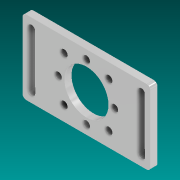
# Autodesk Inventor part: mounting plate stepper motor base 4 mm
Saved by Autodesk Inventor 2020.3 (Build 243373000, 373)
## iProperties
Created: 2020-05-15
Part Number: mounting plate stepper motor base 4 mm
Material: Aluminum 6061
Document SubType Name: Modeling
Designer: Svend
Density: 2.7 g/cm^3
Appearance: Aluminum - Polished
Author: Svend
Autodesk Inventor part; units mm, degrees
ref_plane "YZ Plane" through (0, 0, 0) normal (1, 0, 0) x (0, 1, 0)
ref_plane "XZ Plane" through (0, 0, 0) normal (0, 1, 0) x (-1, 0, 0)
ref_plane "XY Plane" through (0, 0, 0) normal (0, 0, 1) x (1, 0, 0)
sketch "Sketch1" plane through (0, 0, 0) normal (0, 0, 1) x (1, 0, 0)
  circle A0 centre (0, 0) radius 21
  circle A1 centre (16, 0) radius 2
  circle A2 centre (0, 16) radius 2
  circle A3 centre (-16, 0) radius 2
  circle A4 centre (0, -16) radius 2
  line L0 (-14.8492, -14.8492) -> (14.8492, 14.8492)
  line L1 (0, -21) -> (0, 21)
  circle A5 centre (11.3137, 11.3137) radius 1.5
  circle A6 centre (0, 0) radius 12.6
  line L2 (-36.25, -21) -> (36.25, -21)
  line L3 (36.25, 21) -> (-36.25, 21)
  line L4 (-21, -21) -> (21, 21) construction
  line L5 (21, -21) -> (-21, 21) construction
  line L6 (-36.25, 21) -> (-36.25, -21)
  line L7 (36.25, 21) -> (36.25, -21)
  line L8 (-33.35, 17.5) -> (-29.15, 17.5)
  line L9 (-29.15, 17.5) -> (-29.15, -17.5)
  line L10 (-29.15, -17.5) -> (-33.35, -17.5)
  line L11 (-33.35, -17.5) -> (-33.35, 17.5)
  line L12 (-33.35, 17.5) -> (-29.15, -17.5) construction
  line L13 (-29.15, 17.5) -> (-33.35, -17.5) construction
  line L14 (29.15, 17.5) -> (33.35, 17.5)
  line L15 (33.35, 17.5) -> (33.35, -17.5)
  line L16 (33.35, -17.5) -> (29.15, -17.5)
  line L17 (29.15, -17.5) -> (29.15, 17.5)
  line L18 (29.15, 17.5) -> (33.35, -17.5) construction
  line L19 (33.35, 17.5) -> (29.15, -17.5) construction
  line L20 (-26.25, 21) -> (-26.25, -21)
  line L21 (26.25, 21) -> (26.25, -21)
  circle A7 centre (-12.7279, -12.7279) radius 1.621 projected
  circle A8 centre (0, 0) radius 12.5 projected
  circle A9 centre (-12.7279, -12.7279) radius 2 projected
  circle A10 centre (12.7279, 12.7279) radius 2 projected
  circle A11 centre (-12.7279, 12.7279) radius 2 projected
  circle A12 centre (12.7279, -12.7279) radius 2 projected
  circle A13 centre (16, 0) radius 1.6 projected
  circle A14 centre (-16, 0) radius 1.6 projected
  circle A15 centre (0, 16) radius 1.6 projected
  circle A16 centre (0, -16) radius 1.6 projected
  circle A17 centre (0, 0) radius 20.7 projected
  point P0 (-18.984, 8.9782)
  point P1 (-18.984, -8.9782)
  point P2 (-31.25, 0)
  point P3 (31.25, 0)
  point P4 (-31.25, 0)
  point P5 (31.25, 0)
  point P6 (31.25, 0)
  point P7 (31.25, 21)
  point P8 (-31.25, 0)
  point P9 (-31.25, 21)
  point P10 (31.25, 21)
  point P11 (0, 21)
  point P12 (0, -21)
  dimension "d0" = 42
  dimension "d1" = 4
  dimension "d5" = 16
  dimension "d8" = 360
  dimension "d10" = 45
  dimension "d11" = 3
  dimension "d12" = 16
  dimension "d19" = 25.2
  dimension "d31" = 4.2
  dimension "d32" = 35
  dimension "d33" = 4.2
  dimension "d38" = 5
  dimension "d39" = 5
  dimension "d40" = 72.5
  dimension "d41" = 10
  dimension "d42" = 10
  constraints: 42 end point, 17 midpoint, 7 centre point, 6 point on circle, 6 point on line, 5 horizontal alignment, 4 coincident, 4 horizontal, 4 parallel, 3 vertical alignment, 2 perpendicular, 1 tangent, 1 vertical, 20 other
  measures "d0" diameter of A0
  measures "d1" diameter of A1
  measures "d5" distance of point (0, 0) A1.centre
  measures "d10" angle of L1 L0
  measures "d11" diameter of A5
  measures "d12" distance of point (0, 0) A5.centre
  measures "d19" diameter of A6
  measures "d31" distance of L9.end L10.end
  measures "d32" distance of L8.end L9.end
  measures "d33" distance of L15.end L16.end
  measures "d38" distance of L6.start point (-31.25, 21)
  measures "d39" distance from line of L7 point (31.25, 21)
  measures "d40" distance between parallel lines of L6 L7
  measures "d41" distance between parallel lines of L21 L7
  measures "d42" distance between parallel lines of L6 L20
extrude "Extrusion1" add sketch "Sketch1" along normal blind 4 contours A0 L1 A17 L0 | A0 L3 L21 L2 | L0 A17 L1 A0 | L2 L20 L3 A0 | A0 L0 A17 L1 | L1 A17 L0 A0 | A17 L1 A4 A6 L0 A5 A10 | L0 A10 A5 A6 L1 A2 A17 | A17 L0 A9 A6 L1 A4 | L2 L6 L3 L20 | L21 L3 L7 L2 | L1 A2 A6 L0 A9 A17 | A10 L0 A5 | A10 A5 L0 picked at (10.8037, 11.1549) picked at (11.1549, 10.8037)
fillet "Fillet1" radius 2 4 edges at (-36.25, 21, 2) (-36.25, -21, 2) (36.25, -21, 2) (36.25, 21, 2)
fillet "Fillet2" radius 2.1 8 edges at (33.35, -17.5, 2) (29.15, -17.5, 2) (29.15, 17.5, 2) (33.35, 17.5, 2) (-33.35, 17.5, 2) (-29.15, 17.5, 2) (-29.15, -17.5, 2) (-33.35, -17.5, 2)
equation "\"d39\" = d38"
equation "\"d42\" = d41"
body "Solid1"
